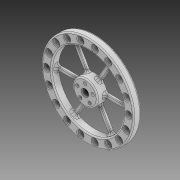
# Autodesk Inventor part: Flywheel
Saved by Autodesk Inventor 2020 (Build 240168000, 168)
## iProperties
Created: 2020-12-31
Part Number: Flywheel
Material: Generic
Document SubType Name: Modeling
Designer: DDeGo
Density: 1 g/cm^3
Appearance: Default
Author: DDeGo
Autodesk Inventor part; units mm, degrees
ref_plane "YZ Plane" through (0, 0, 0) normal (1, 0, 0) x (0, 1, 0)
ref_plane "XZ Plane" through (0, 0, 0) normal (0, 1, 0) x (-1, 0, 0)
ref_plane "XY Plane" through (0, 0, 0) normal (0, 0, 1) x (1, 0, 0)
sketch "Sketch2" plane through (0, 0, 0) normal (0, 0, 1) x (1, 0, 0)
  circle A0 centre (0, 0) radius 1.55
  circle A1 centre (0, 0) radius 10
  dimension "d46" = 20
  dimension "d47" = 3.1
  constraints: 2 centre point, 1 coincident
  measures "d46" diameter of A1
  measures "d47" diameter of A0
extrude "Extrusion2" add sketch "Sketch2" along normal blind 8
sketch "Sketch6" plane through (0, 0, 0) normal (0, 0, -1) x (-1, 0, 0)
  circle A0 centre (0, 0) radius 29.5
  circle A1 centre (0, 0) radius 37.5
  dimension "d23" = 75
  dimension "d24" = 8
  constraints: 2 centre point, 2 coincident
  measures "d23" diameter of A1
  measures "d24" radial gap between concentric circles of A0 A1
extrude "Extrusion6" add sketch "Sketch6" against normal blind 6
sketch "Sketch7" plane through (0, 0, 0) normal (0, 0, -1) x (-1, 0, 0)
  line L0 (-3.6444, 9.3123) -> (-13.4319, 26.2647)
  circle A0 centre (0, 0) radius 29.5 projected
  line L1 (-13.4319, 26.2647) -> (-16.03, 24.7647) construction
  line L2 (-16.03, 24.7647) -> (-6.2425, 7.8123)
  line L3 (-6.2425, 7.8123) -> (-3.6444, 9.3123) construction
  line L4 (0, 0) -> (0, 10) construction
  circle A1 centre (0, 0) radius 10 projected
  point P0 (-3.6444, 9.3123)
  dimension "d28" = 3
  dimension "d48" = 30
  constraints: 10 end point, 4 point on circle, 3 perpendicular, 1 vertical
  measures "d28" distance between parallel lines of L0 L2
  measures "d48" angle of L0 L4
extrude "Extrusion7" add sketch "Sketch7" against normal blind 2 contours A1 L2 A0 L0 picked at (-8.1007, 14.3643)
fillet "Fillet1" radius 2 6 edges at (13.4319, 26.2647, 1) (16.03, 24.7647, 1) (14.75, 25.5477, 2) (5, 8.6603, 2) (6.2425, 7.8123, 1) (3.6444, 9.3123, 1)
fillet "Fillet1" radius 0.5 2 edges at (11.1362, 16.2885, 2) (8.5381, 17.7885, 2)
pattern_circular "Circular Pattern1" count 6 over 360 about axis through (0, 0, 0) along (0, 0, 1) of "Extrusion7", "Fillet1"
sketch "Sketch8" plane through (0, 0, 6) normal (0, 0, 1) x (1, 0, 0)
  circle A0 centre (0, 0) radius 37.5 projected
  line L0 (37.5, 0) -> (29.5, 0) construction
  circle A1 centre (33.5, 0) radius 2.5
  circle A2 centre (0, 0) radius 29.5 projected
  dimension "d37" = 5
  constraints: 2 end point, 2 horizontal alignment, 1 centre point, 1 horizontal, 1 midpoint, 1 point on line, 2 other
  measures "d37" diameter of A1
extrude "Extrusion8" cut sketch "Sketch8" against normal through all contours A1
chamfer "Chamfer1" distance 0.5 angle 45 1 edges at (31, 0, 6)
pattern_circular "Circular Pattern2" count 18 over 360 about axis through (0, 0, 0) along (0, 0, 1) of "Extrusion8", "Chamfer1"
fillet "Fillet2" radius 1 4 edges at (29.5, 0, 6) (37.5, 0, 6) (37.5, 0, 0) (-10, 0, 8)
sketch "Sketch10" plane through (0, 0, 0) normal (0, 0, -1) x (-1, 0, 0)
  circle A0 centre (0, 0) radius 2.6
  dimension "d53" = 5.2
  constraints: 1 centre point, 1 coincident
  measures "d53" diameter of A0
extrude "Extrusion10" cut sketch "Sketch10" against normal blind 2
sketch "Sketch11" plane through (0, 0, 8) normal (0, 0, 1) x (1, 0, 0)
  circle A0 centre (0, 0) radius 3
  dimension "d56" = 6
  constraints: 1 centre point, 1 coincident
  measures "d56" diameter of A0
extrude "Extrusion11" cut sketch "Sketch11" against normal blind 4
chamfer "Chamfer2" distance 1 angle 45 1 edges at (-1.55, 0, 2)
sketch "Sketch12" plane through (0, 0, 8) normal (0, 0, 1) x (1, 0, 0)
  circle A0 centre (0, 0) radius 10 projected
  line L0 (0, 10) -> (0, 3) construction
  circle A1 centre (0, 0) radius 3 construction
  line L1 (0, 0) -> (0, 3) construction
  circle A2 centre (0, 6.5) radius 1.35
  circle A3 centre (-6.1819, 2.0086) radius 1.35
  circle A4 centre (-3.8206, -5.2586) radius 1.35
  circle A5 centre (3.8206, -5.2586) radius 1.35
  circle A6 centre (6.1819, 2.0086) radius 1.35
  dimension "d62" = 2.7
  dimension "d65" = 360
  constraints: 5 centre point, 4 end point, 2 vertical alignment, 1 collinear, 1 midpoint, 1 vertical, 13 other
  measures "d62" diameter of A2
extrude "Extrusion12" cut sketch "Sketch12" against normal through all contours A2 | A3 | A4 | A5 | A6
body "Solid2"
